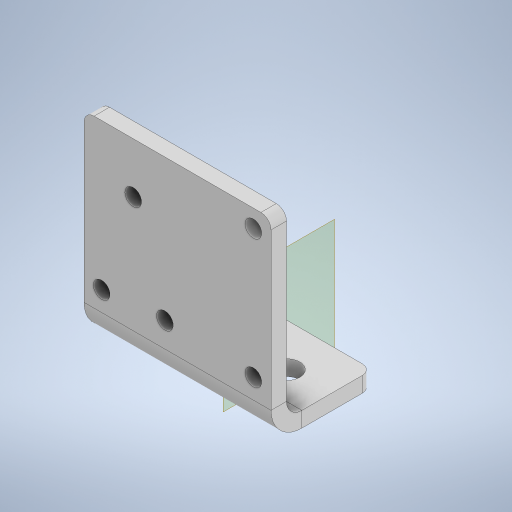
# Autodesk Inventor part: XY Idler Mount
Saved by Autodesk Inventor 2024 (Build 280153000, 153)
## iProperties
Created: 2024-12-28
Part Number: XY Idler Mount
Material: Generic
Document SubType Name: Sheet Metal
Designer: Ishaan
Density: 1 g/cm^3
Appearance: Default
Sheet Metal Rule: Default
Author: Ishaan
Autodesk Inventor part; units mm, degrees
ref_plane "YZ Plane" through (0, 0, 0) normal (1, 0, 0) x (0, 1, 0)
ref_plane "XZ Plane" through (0, 0, 0) normal (0, 1, 0) x (-1, 0, 0)
ref_plane "XY Plane" through (0, 0, 0) normal (0, 0, 1) x (1, 0, 0)
sketch "Sketch1" plane through (0, 0, 0) normal (0, 0, 1) x (1, 0, 0)
  line L0 (18.5, -19.5) -> (-18.5, -19.5)
  line L1 (-18.5, -19.5) -> (-18.5, 19.5)
  line L2 (-18.5, 19.5) -> (18.5, 19.5)
  line L3 (18.5, 19.5) -> (18.5, -19.5)
  line L4 (18.5, -19.5) -> (-18.5, 19.5) construction
  line L5 (-18.5, -19.5) -> (18.5, 19.5) construction
  circle A0 centre (-2.5, -8.5) radius 9 construction
  circle A1 centre (-8.764, 9.5) radius 9 construction
  circle A2 centre (-15, -9.5) radius 2.5 construction
  circle A3 centre (15, 16) radius 2.5 construction
  circle A4 centre (15, -9.5) radius 2.5 construction
  line L6 (-15, -9.5) -> (15, -9.5) construction
  point P0 (0, 0)
  point P1 (0, -9.5)
  dimension "d0" = 37
  dimension "d1" = 39
  dimension "d2" = 11
  dimension "d3" = 2.5
  dimension "d4" = 18
  dimension "d5" = 18
  dimension "d6" = 18
  dimension "d7" = 6.264
  dimension "d8" = 5
  dimension "d10" = 30
  dimension "d11" = 10
  dimension "d12" = 3.5
  dimension "d13" = 3.5
  constraints: 14 end point, 5 centre point, 5 coincident, 3 midpoint, 2 equal radius, 2 horizontal, 2 parallel, 2 vertical alignment, 1 perpendicular
  measures "d0" distance of L1.end L2.end
  measures "d1" distance of L0.end L1.end
  measures "d2" distance from line of L0 point (-2.5, -8.5)
  measures "d3" horizontal distance of point (0, 0) point (-2.5, -8.5)
  measures "d4" diameter of A0
  measures "d5" diameter of A1
  measures "d6" vertical distance of A0.centre A1.centre
  measures "d7" horizontal distance of A0.centre A1.centre
  measures "d8" diameter of A2
  measures "d10" distance of L6.start L6.end
  measures "d11" distance between parallel lines of L0 L6
  measures "d12" distance from line of L3 A3.centre
  measures "d13" distance from line of L2 A3.centre
extrude "Plate1" add sketch "Sketch1" along normal blind 3.048
sketch "Sketch2" plane through (-18.5, -16.452, 3.048) normal (0, -1, 0) x (1, 0, 0)
  line L0 (37, 0) -> (0, 0)
  line L1 (0, 0) -> (0, -20.048)
  line L2 (0, -20.048) -> (37, -20.048)
  line L3 (37, -20.048) -> (37, 0)
  constraints: 6 end point, 1 horizontal, 1 perpendicular, 1 vertical
edge flange "Flange1" height 17 angle 90 thickness 3.048 bend radius 3.048 thickness toward (0, -1, 0) relief tear relief width 3.048 relief depth 1.524 edges at (0, -19.5, 0) wall of the first edge with corners at (18.5, -16.452, 3.048) (-18.5, -16.452, 3.048) (-18.5, -16.452, -17) (18.5, -16.452, -17)
bend "Bend1"
corner "Corner1"
hole "Hole1" at (-2.5, -8.5, 0) at (-8.764, 9.5, 0) direction (0, 0, 1) diameter 3.3 end through all
hole "Hole2" at (15, 16, 0) at (15, -9.5, 0) at (-15, -9.5, 0) direction (0, 0, 1) diameter 3.3 end through all
sketch "Sketch3" plane through (-18.5, -16.452, -17) normal (0, 1, 0) x (1, 0, 0)
  line L0 (0, -13.952) -> (37, -13.952) construction
  line L1 (37, -13.952) -> (37, 0) construction
  line L2 (37, 0) -> (0, 0) construction
  line L3 (0, -13.952) -> (0, 0) construction
  line L4 (8.5, -8.5) -> (28.5, -8.5) construction
  line L5 (8.5, -8.5) -> (0, -8.5) construction
  line L6 (0, -8.5) -> (0, 0) construction
  line L7 (0, 0) -> (8.5, 0) construction
  line L8 (8.5, 0) -> (8.5, -8.5) construction
  point P0 (18.5, -17)
  point P1 (18.5, 0)
  point P2 (18.5, -8.5)
  dimension "d39" = 20
  constraints: 10 end point, 2 coincident, 2 horizontal, 2 midpoint, 2 parallel, 2 perpendicular, 1 vertical alignment
  measures "d39" distance of L4.start L4.end
hole "Hole3" at (-10, -16.452, -8.5) at (10, -16.452, -8.5) direction (0, -1, 0) diameter 5.3 end through all
fillet "Fillet1" radius 2 4 edges at (18.5, -17.976, -17) (-18.5, 19.5, 1.524) (18.5, 19.5, 1.524) (-18.5, -17.976, -17)
ref_plane "Work Plane1" through (0, -16.452, -17) normal (-1, 0, 0) x (0, -1, 0)
equation "\"d13\" = d12"
equation "\"d30\" = Thickness"
equation "\"d14\" = Thickness"
equation "\"d15\" = BendReliefWidth"
equation "\"d16\" = BendReliefDepth"
equation "\"d17\" = MinimumRemnant"
equation "\"d18\" = TransitionRadius"
equation "\"d21\" = BendRadius"
equation "\"d22\" = CornerReliefSize"
equation "\"d23\" = GapSize"
equation "\"d24\" = JacobiRadiusSize"
equation "\"BendRadius\" = Thickness"
equation "\"BendReliefWidth\" = Thickness"
equation "\"BendReliefDepth\" = 0.5 * Thickness"
equation "\"CornerReliefSize\" = 4 * Thickness"
equation "\"MinimumRemnant\" = 2 * Thickness"
equation "\"TransitionRadius\" = BendRadius"
equation "\"JacobiRadiusSize\" = BendRadius"
equation "\"GapSize\" = Thickness"
equation "\"Thickness\" = 3.048"
body "Solid1"
